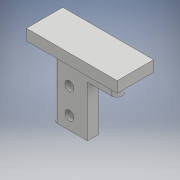
# Autodesk Inventor part: StartSupport
Saved by Autodesk Inventor 2018 (Build 220112000, 112)
## iProperties
Created: 2020-05-13
Part Number: StartSupport
Material: Generic
Document SubType Name: Modeling
Designer: Ivan
Density: 1 g/cm^3
Appearance: Default
Author: Ivan
Autodesk Inventor part; units mm, degrees
ref_plane "YZ Plane" through (0, 0, 0) normal (1, 0, 0) x (0, 1, 0)
ref_plane "XZ Plane" through (0, 0, 0) normal (0, 1, 0) x (-1, 0, 0)
ref_plane "XY Plane" through (0, 0, 0) normal (0, 0, 1) x (1, 0, 0)
sketch "Sketch1" plane through (0, 0, 0) normal (0, 0, 1) x (1, 0, 0)
  line L0 (7.5, -1.5) -> (-7.5, -1.5)
  arc A0 (7.5, -1.5) -> (7.5, 1.5) centre (7.3777, 0) ccw
  line L1 (0, -2.1) -> (0, 2.1) construction
  arc A1 (-7.5, 1.5) -> (-7.5, -1.5) centre (-7.3777, 0) ccw
  line L2 (-12.4357, 0) -> (12.4357, 0) construction
  line L3 (7.5, 1.5) -> (-7.5, 1.5)
  point P0 (0, 0)
  point P1 (0, 1.5)
  dimension "d0" = 15
  dimension "d1" = 3
  constraints: 4 end point, 4 point on circle, 2 centre point, 2 symmetric about line, 1 coincident, 1 horizontal alignment, 1 vertical alignment, 1 other
  measures "d0" distance of L0.start L0.end
  measures "d1" distance of L3.start L0.start
extrude "Extrusion1" add sketch "Sketch1" along normal blind 4.95
sketch "Sketch2" plane through (0, 0, 4.95) normal (0, 0, 1) x (1, 0, 0)
  line L0 (-12.5, 5) -> (12.5, 5)
  line L1 (12.5, 5) -> (12.5, -5)
  line L2 (12.5, -5) -> (-12.5, -5)
  line L3 (-12.5, -5) -> (-12.5, 5)
  point P0 (0, 0)
  point P1 (0, 5)
  point P2 (12.5, 0)
  dimension "d4" = 25
  dimension "d5" = 10
  constraints: 8 end point, 2 midpoint, 2 parallel, 1 horizontal, 1 horizontal alignment, 1 perpendicular, 1 vertical alignment
  measures "d4" distance of L1.end L2.end
  measures "d5" distance of L0.end L1.end
extrude "Extrusion2" add sketch "Sketch2" along normal blind 3
sketch "Sketch3" plane through (0, 0, 0) normal (0, 0, -1) x (-1, 0, 0)
  line L0 (-0.8, 1.5) -> (-0.8, -1.5)
  line L1 (-0.8, -1.5) -> (7.5, -1.5)
  arc A0 (7.5, -1.5) -> (7.5, 1.5) centre (7.3777, 0) ccw projected
  line L2 (7.5, 1.5) -> (-0.8, 1.5)
  line L3 (7.5, 1.5) -> (-7.5, 1.5) projected
  point P0 (0, 0)
  constraints: 6 end point, 1 horizontal, 1 point on line
extrude "Extrusion3" add sketch "Sketch3" along normal blind 14
sketch "Sketch5" plane through (-7.5, 1.5, 4.95) normal (0, 1, 0) x (1, 0, 0)
  circle A0 centre (3.35, 8.35) radius 1.25
  circle A1 centre (3.35, 15.374) radius 1.25
  line L0 (-5, 0) -> (-5, -3) projected
  line L1 (-5, 0) -> (20, 0) projected
  point P0 (7.5, 4.95)
  dimension "d18" = 2.5
  dimension "d19" = 8.35
  dimension "d20" = 8.35
  dimension "d21" = 7.024
  constraints: 2 centre point, 1 equal radius, 1 vertical alignment
  measures "d18" diameter of A0
  measures "d19" distance from line of L0 A0.centre
  measures "d20" distance from line of L1 A0.centre
  measures "d21" distance of A1.centre A0.centre
extrude "Extrusion5" cut sketch "Sketch5" against normal through all
body "Solid1"
